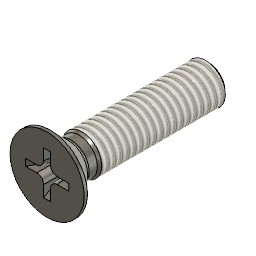
full file (Autodesk Fusion 360 archive; units mm, degrees)
design "Countersunk Flat Head Screw NF EN ISO 7046-1 - M3 x 12 - H Steel 4.6 Plain"
description: Countersunk Flat Head Screw NF EN ISO 7046-1 - M3 x 12 - H
part number: NF EN ISO 7046-1 - M3 x 12 - H Steel 4.6 Plain
Autodesk Fusion 360 part; units mm, degrees
sketch "Sketch1" plane through (0, 0, 0) normal (0, 1, 0) x (1, 0, 0)
  line L0 (0, -2.9966) -> (-2.75, -2.9966)
  line L1 (-2.75, -2.9966) -> (-2.75, -2.75)
  line L2 (-2.75, -2.75) -> (-1.3466, -1.3466)
  line L3 (-1.5, -0.3466) -> (-1.5, 9.0034)
  line L4 (-1.5, 9.0034) -> (0, 9.0034)
  line L5 (0, 9.0034) -> (0, -2.9966)
  line L6 (-1.3466, -0.6123) -> (-1.3466, -1.3466)
  line L7 (-1.5, -0.3466) -> (-1.3466, -0.6123)
  dimension "d9" = 3
  dimension "d11" = 5.5
  dimension "d71" = 1.65
  dimension "d72" = 2.6933
  dimension "d89" = 9.35
  dimension "d101" = 30
  dimension "d115" = 12
  dimension "d121" = 45
  constraint perpendicular L0 L1
  constraint vertical L3
  constraint perpendicular L3 L4
  constraint perpendicular L0 L5
  constraint collinear origin L0.start L4.end
  constraint horizontal L0
  constraint coincident L2.end L6.end
  constraint coincident L6 L7.end
  constraint coincident L6.start L7.end
  constraint coincident origin L2
  measures "d71" distance of L0 L2.end
  measures "d89" distance of L4 L3.start
  measures "d101" angle of L3 L7
  measures "d115" distance of L0.start L4
  measures "d121" angle of L2 L5
revolve "Revolve1" add sketch "Sketch1" angle 360 about axis through (0, 0, -9.0034) along (0, 0, 1) makes body 1
sketch "Sketch2" plane through (0, 0, 2.9966) normal (0, 0, 1) x (1, 0, 0)
  line L0 (-0.255, 0.255) -> (-1.6, 0.255)
  line L1 (-1.6, 0.255) -> (-1.6, -0.255)
  line L2 (-1.6, -0.255) -> (-0.255, -0.255)
  line L3 (0.255, -1.6) -> (0.255, -0.255)
  line L4 (-0.255, -1.6) -> (0.255, -1.6)
  line L5 (-0.255, -0.255) -> (-0.255, -1.6)
  line L6 (1.6, 0.255) -> (0.255, 0.255)
  line L7 (1.6, -0.255) -> (1.6, 0.255)
  line L8 (0.255, -0.255) -> (1.6, -0.255)
  line L9 (-0.255, 1.6) -> (-0.255, 0.255)
  line L10 (0.255, 1.6) -> (-0.255, 1.6)
  line L11 (0.255, 0.255) -> (0.255, 1.6)
  dimension "d111" = 360
  dimension "d117" = 3.2
  dimension "d122" = 0.51
  constraint horizontal L0
  constraint perpendicular L0 L1
  constraint vertical L0.start L2.end
  constraint coincident L0.start L9.end
  measures "d117" distance of L4.start L10
  measures "d122" distance of L0 L2
extrude "Extrude1" add sketch "Sketch2" against normal blind 2.1 draft -4 separate body makes body 2
draft "Draft1" angle -30 neutral plane through (0, 0, 2.9966) pull (0, 0, 1) 4 faces at (1.5511, 0.0361, 2.2966) (0.0361, 1.5511, 2.2966) (-1.5511, -0.0361, 2.2966) (0.0361, -1.5511, 2.2966) on bodies 2
fillet "Fillet3" radius 0.51 4 edges at (0.1816, 0.1816, 1.9466) (0.1816, -0.1816, 1.9466) (-0.1816, -0.1816, 1.9466) (-0.1816, 0.1816, 1.9466) on bodies 2
combine "Combine1" operation cut target body 1 tool bodies 2
thread "Thread1" "ISO Metric profile 3.0 M3x0.5 M3x0.5 6g" major diameter 2.927 minor diameter 2.3555 pitch 0.5 angle 60 resizes the face on face at (-1.4981, 0.0748, -2.77) on bodies 1
fillet "Fillet5" radius 0.3 1 edges at (-1.2555, 0.487, 1.3466) on bodies 1
sketch "Sketch6" plane through (0, 0, 0) normal (0, 1, 0) x (1, 0, 0)
  line L0 (-1.1933, 9.0034) -> (-1.53, 9.0034)
  line L1 (-1.53, 9.0034) -> (-1.53, 8.6966)
  line L2 (-1.53, 8.6966) -> (-1.1933, 9.0034)
  line L3 (-1.5, 9.0034) -> (0, 9.0034)
  line L4 (0, 0) -> (0, 9.0034) construction
  dimension "d102" = 1.53
  dimension "d118" = 1.1933
  dimension "d119" = 0.3067
  constraint horizontal L0
  constraint perpendicular L0 L1
  constraint coincident L0.start L3
  constraint coincident L4.start origin
  constraint coincident L3.end L4.end
  measures "d102" distance of L4.start L1
  measures "d118" distance of L0.start L4
  measures "d119" distance of L0 L1.end
revolve "Revolve3" cut sketch "Sketch6" angle 360 about axis through (0, 0, 1.75) along (0, 0, 1) bodies 1
equation "d9 = adsk_nomdia"
equation "d11 = adsk_headdia"
equation "adsk_nomlen = 12.00 mm"
equation "adsk_headh = 1.65 mm"
equation "adsk_headdia = 5.50 mm"
equation "adsk_nomdia = 3.00 mm"
equation "adsk_headang = 90.00 deg"
equation "adsk_phildia = 3.20 mm"
equation "d31 = -adsk_phildepth"
equation "adsk_philwidth = 0.51 mm"
equation "adsk_phildepth = 2.10 mm"
equation "d71 = adsk_headh"
equation "d72 = adsk_shnkdia"
equation "adsk_shnkdia = 2.693275 mm"
equation "d89 = adsk_thrlen"
equation "adsk_thrlen = 9.35 mm"
equation "adsk_pitch1 = 0.50 mm"
equation "adsk_startlen = 0.306725 mm"
equation "adsk_midfillet = adsk_nomdia * 0.1"
equation "d96 = adsk_midfillet"
equation "d99 = ( adsk_shnkdia / 2 ) * tan(90 deg - adsk_headang / 2) + adsk_headh"
equation "d102 = adsk_nomdia * 0.51"
equation "adsk_endpointdia = 2.38655 mm"
equation "d114 = adsk_philwidth"
equation "d115 = adsk_nomlen"
equation "d117 = adsk_phildia"
equation "d118 = adsk_endpointdia / 2"
equation "d119 = adsk_startlen"
equation "d121 = adsk_headang * 0.5"
equation "d122 = adsk_philwidth"
